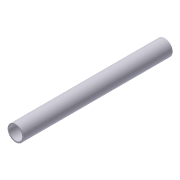
# Autodesk Inventor part: FE-00006-03
Saved by Autodesk Inventor 2012 (Build 160160000, 160)
## iProperties
Created: 2008-05-24
Part Number: FE-00006-03
Document SubType Name: Modeling
Designer: firstuser
Density: 1 g/cm^3
Mass: 169.692 g
Surface Area: 961.06 cm^2
Volume: 169.692 cm^3
Material: Default
Author: firstuser
Autodesk Inventor part; units mm, degrees
ref_plane "YZ Plane" through (0, 0, 0) normal (1, 0, 0) x (0, 1, 0)
ref_plane "XZ Plane" through (0, 0, 0) normal (0, 1, 0) x (-1, 0, 0)
ref_plane "XY Plane" through (0, 0, 0) normal (0, 0, 1) x (1, 0, 0)
sketch "Sketch1" plane through (0, 0, 0) normal (0, 0, 1) x (1, 0, 0)
  circle A0 centre (0, 0) radius 21.0312
  circle A1 centre (0, 0) radius 17.4625
  dimension "d0" = 42.0624
  dimension "d1" = 34.925
  constraints: 2 centre point, 1 coincident
  measures "d0" diameter of A0
  measures "d1" diameter of A1
extrude "Extrusion1" add sketch "Sketch1" along normal blind 393.7
sketch "Sketch2" plane through (0, 0, 0) normal (0, 1, 0) x (-1, 0, 0)
  line L0 (0, -78.74) -> (0, 472.44) projected
  line L1 (-21.0312, 393.7) -> (21.0312, 393.7) projected
  line L2 (-21.0312, 0) -> (21.0312, 0) projected
  line L3 (21.0312, 0) -> (21.0312, 393.7) projected
  line L4 (-21.0312, 0) -> (21.0312, 0) projected
  circle A0 centre (0, 31.75) radius 3.175
  circle A1 centre (0, 82.55) radius 3.175
  dimension "d4" = 6.35
  dimension "d5" = 50.8
  dimension "d6" = 31.75
  constraints: 2 centre point, 2 point on line, 1 equal radius
  measures "d4" diameter of A1
  measures "d5" distance of A0.centre A1.centre
  measures "d6" distance from line of L2 A0.centre
extrude "Extrusion2" cut sketch "Sketch2" along normal through all contours A0 L0 | L0 A0 | A1 L0 | L0 A1
body "Solid1"
